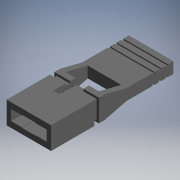
# Autodesk Inventor part: SNT-100-BK-H_body
Saved by Autodesk Inventor 2017.3 (Build 213256000, 256)
## iProperties
Part Number: SNT-100-BK-H_body
Material: Generic
Catalog Web Link: www.cadenas.de
Description: SNT Body-SNT Series - (2,54 mm) .100" Shunt
Vendor: SAMTEC
Document SubType Name: Modeling
Designer: partserver
Manufacturer: SAMTEC
Mass: 0.0856152 g
Surface Area: 2.94335 cm^2
Volume: 0.0856152 cm^3
Density: 1 g/cm^3
Appearance: PSOLRGB-127-127-127
Category: PARTsolutions
Company: SAMTEC
Title: SNT-100-BK-H_body
Author: Cadenas PARTsolutions
Comments: SNT Series - (2,54 mm) .100" Shunt
PSOL_IDENT_0: {$CADENAS_DATA\23d-libs\samtec\modelling\snt\parts\snt_body.prj},186 {VTYP=3D},{NB=SNT-100-BK-H_body
PSOL_IDENT_1: },{LINA=SNT-100-BK-H_body},{NN=SNT Body},{DATE=12.08.2019 09:26:17},{GEOMDATE=12.06.2019 10:29:52},{
PSOL_IDENT_2: VERSION=},{LINEID=10},{WBVAR=COLOR,HOPT},{WBNUMERIC=}  {NB=SNT-100-BK-H_body},{LINA=SNT-100-BK-H_bod
PSOL_IDENT_3: y},{KT=DUMMY},{PN=SNT-100-BK-H},{SERIES=SNT},{COLOR=BK},{HOPTALG=   ''  , 'Not Selected' , 'H' , 'Ha
PSOL_IDENT_4: ndle'  },{HOPT=H},{A=0.240},{W=0.100},{L=0.200},{PINW=0.040},{HPN=-H},{COL=0.50,0.50,0.50,0.00}
NB: SNT-100-BK-H_body
NN: SNT Body
NT: SNT Series - (2,54 mm) .100" Shunt
NBSYN: $PN._body
LINA: SNT-100-BK-H_body
CATALOG: Samtec
PN: SNT-100-BK-H
SERIES: SNT
COLOR: Black
HOPT: Handle
A: 0.24
W: 0.1
L: 0.2
PINW: 0.04
SUPPLIER: SAMTEC
ARTICLENO: SNT-100-BK-H_body
BOMINFO: SNT-100-BK-H_body
CREATOR: CADENAS GmbH
Autodesk Inventor part; units mm, degrees
sketch "Sketch_1" plane through (0, 0, 0) normal (0, 1, 0) x (1, 0, 0)
  line L0 (-2.54, 1.27) -> (-2.54, -1.27)
  line L1 (-2.54, -1.27) -> (2.54, -1.27)
  line L2 (2.54, -1.27) -> (2.54, 1.27)
  line L3 (2.54, 1.27) -> (-2.54, 1.27)
  constraints: 8 end point
extrude "Extrusion1" add sketch "Sketch_1" along normal blind 6.096
sketch "Sketch_2" plane through (0, 5.461, 0) normal (0, 1, 0) x (1, 0, 0)
  line L0 (-2.794, 2.54) -> (-2.794, -2.54)
  line L1 (-2.794, -2.54) -> (2.794, -2.54)
  line L2 (2.794, -2.54) -> (2.794, 2.54)
  line L3 (2.794, 2.54) -> (-2.794, 2.54)
  line L4 (-2.286, 1.016) -> (-2.286, -1.016)
  line L5 (-2.286, -1.016) -> (2.286, -1.016)
  line L6 (2.286, -1.016) -> (2.286, 1.016)
  line L7 (2.286, 1.016) -> (-2.286, 1.016)
  constraints: 16 end point
extrude "Extrusion2" cut sketch "Sketch_2" against normal blind 0.508
sketch "Sketch_3" plane through (0, 6.096, 0) normal (0, 1, 0) x (1, 0, 0)
  line L0 (-0.762, 1.27) -> (-0.762, -1.27)
  line L1 (-0.762, -1.27) -> (0.762, -1.27)
  line L2 (0.762, -1.27) -> (0.762, 1.27)
  line L3 (0.762, 1.27) -> (-0.762, 1.27)
  constraints: 8 end point
extrude "Extrusion3" cut sketch "Sketch_3" against normal blind 2.54
sketch "Sketch_4" plane through (0, 6.096, 0) normal (0, 1, 0) x (1, 0, 0)
  line L0 (-1.778, 0.4445) -> (-1.778, -0.4445)
  line L1 (-1.778, -0.4445) -> (1.778, -0.4445)
  line L2 (1.778, -0.4445) -> (1.778, 0.4445)
  line L3 (1.778, 0.4445) -> (-1.778, 0.4445)
  constraints: 8 end point
extrude "Extrusion4" cut sketch "Sketch_4" against normal blind 6.096
sketch "Sketch_5" plane through (0, 5.7912, 0) normal (0, 1, 0) x (1, 0, 0)
  line L0 (-2.032, 0.5969) -> (-2.032, -0.5969)
  line L1 (-2.032, -0.5969) -> (2.032, -0.5969)
  line L2 (2.032, -0.5969) -> (2.032, 0.5969)
  line L3 (2.032, 0.5969) -> (-2.032, 0.5969)
  constraints: 8 end point
extrude "Extrusion5" cut sketch "Sketch_5" against normal blind 6.096
sketch "Sketch_8" plane through (0, 0, 0) normal (0, 1, 0) x (-1, 0, 0)
  line L0 (0.762, -0.6477) -> (0.762, 0.6477)
  line L1 (0.762, 0.6477) -> (-0.762, 0.6477)
  line L2 (-0.762, 0.6477) -> (-0.762, -0.6477)
  line L3 (-0.762, -0.6477) -> (0.762, -0.6477)
  constraints: 8 end point
extrude "Extrusion6" cut sketch "Sketch_8" along normal blind 3.556
sketch "Sketch_6" plane through (0, 0, 0) normal (1, 0, 0) x (0, 1, 0)
  line L0 (3.0093, 0.2159) -> (2.2752, -0.6477)
  line L1 (2.2752, -0.6477) -> (6.096, -0.6477)
  line L2 (6.096, -0.6477) -> (6.096, 0.2159)
  line L3 (6.096, 0.2159) -> (3.0093, 0.2159)
  constraints: 8 end point
extrude "Extrusion7" add sketch "Sketch_6" along normal mid plane 1.27
sketch "Sketch_7" plane through (0, 0, 0) normal (1, 0, 0) x (0, 1, 0)
  line L0 (6.096, 1.27) -> (6.096, -1.27)
  line L1 (6.096, -1.27) -> (8.636, -0.635)
  line L2 (8.636, -0.635) -> (11.557, -0.635)
  line L3 (11.557, -0.635) -> (11.557, -0.508)
  line L4 (11.557, -0.508) -> (11.811, -0.508)
  line L5 (11.811, -0.508) -> (11.811, -0.635)
  line L6 (11.811, -0.635) -> (12.319, -0.635)
  line L7 (12.319, -0.635) -> (12.319, -0.508)
  line L8 (12.319, -0.508) -> (12.573, -0.508)
  line L9 (12.573, -0.508) -> (12.573, -0.635)
  line L10 (12.573, -0.635) -> (13.081, -0.635)
  line L11 (13.081, -0.635) -> (13.081, -0.508)
  line L12 (13.081, -0.508) -> (13.335, -0.508)
  line L13 (13.335, -0.508) -> (13.335, -0.635)
  line L14 (13.335, -0.635) -> (13.97, -0.635)
  line L15 (13.97, -0.635) -> (13.97, 0.635)
  line L16 (13.97, 0.635) -> (13.335, 0.635)
  line L17 (13.335, 0.635) -> (13.335, 0.508)
  line L18 (13.335, 0.508) -> (13.081, 0.508)
  line L19 (13.081, 0.508) -> (13.081, 0.635)
  line L20 (13.081, 0.635) -> (12.573, 0.635)
  line L21 (12.573, 0.635) -> (12.573, 0.508)
  line L22 (12.573, 0.508) -> (12.319, 0.508)
  line L23 (12.319, 0.508) -> (12.319, 0.635)
  line L24 (12.319, 0.635) -> (11.811, 0.635)
  line L25 (11.811, 0.635) -> (11.811, 0.508)
  line L26 (11.811, 0.508) -> (11.557, 0.508)
  line L27 (11.557, 0.508) -> (11.557, 0.635)
  line L28 (11.557, 0.635) -> (8.636, 0.635)
  line L29 (8.636, 0.635) -> (6.096, 1.27)
  constraints: 60 end point
extrude "Extrusion8" add sketch "Sketch_7" along normal mid plane 5.08
sketch "Sketch_10" plane through (0, 0, 0) normal (1, 0, 0) x (0, 1, 0)
  line L0 (8.636, 1.27) -> (6.096, 1.27)
  line L1 (6.096, 1.27) -> (6.096, -1.27)
  line L2 (6.096, -1.27) -> (8.636, -1.27)
  line L3 (8.636, -1.27) -> (8.636, 1.27)
  constraints: 8 end point
extrude "Extrusion9" cut sketch "Sketch_10" along normal mid plane 3.81
ref_plane "body_to_dummy_XY" through (0, 0, 0) normal (0, -1, 0) x (1, 0, 0)
ref_plane "body_to_dummy_YZ" through (0, 0, 0) normal (1, 0, 0) x (0, 0, 1)
ref_plane "body_to_dummy_ZX" through (0, 0, 0) normal (0, 0, 1) x (0, -1, 0)
body "Solid1"
